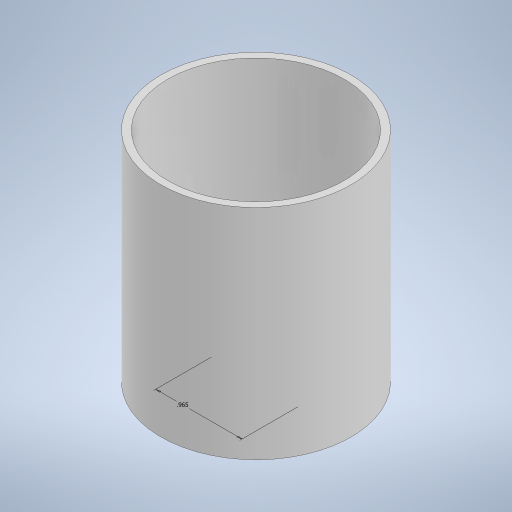
# Autodesk Inventor part: UpstreamVolume
Saved by Autodesk Inventor 2023 (Build 270158000, 158)
## iProperties
Created: 2023-01-27
Part Number: UpstreamVolume
Material: Generic
Document SubType Name: Modeling
Designer: remidm
Density: 1 g/cm^3
Appearance: Default
DistanceBetweenHolesSweep: 0.965 in
Author: remidm
Autodesk Inventor part; units mm, degrees
ref_plane "YZ Plane" through (0, 0, 0) normal (1, 0, 0) x (0, 1, 0)
ref_plane "XZ Plane" through (0, 0, 0) normal (0, 1, 0) x (-1, 0, 0)
ref_plane "XY Plane" through (0, 0, 0) normal (0, 0, 1) x (1, 0, 0)
sketch "Sketch1" plane through (0, 0, 0) normal (0, 0, 1) x (1, 0, 0)
  line L0 (-25, 0) -> (-25, 60)
  line L1 (-27, 60) -> (-27, -2)
  line L2 (-25, 0) -> (0, 0)
  line L3 (0, 0) -> (0, -2)
  line L4 (0, -2) -> (-27, -2)
  line L5 (0, -14.4) -> (0, 72.4) projected
  line L6 (-27, 60) -> (-25, 60)
  dimension "d5" = 2
  dimension "radius" = 25
  dimension "d7" = 2
  constraints: 12 end point, 2 horizontal, 2 perpendicular, 1 vertical
  measures "d5" distance between parallel lines of L4 L2
  measures "radius" distance from line of L2.end L0
  measures "d7" distance between parallel lines of L0 L1
revolve "Revolution1" add sketch "Sketch1" angle 360 about axis through (0, -10, 0) along (0, 1, 0)
sketch "Sketch3" plane through (0, -2, 0) normal (0, -1, 0) x (1, 0, 0)
  point P0 (0, 0)
  point P1 (-12.4915, 0)
  point P2 (12.0084, 0)
  dimension "DistanceBetweenHolesSweep" = 24.5
  measures "DistanceBetweenHolesSweep" distance of point (12.008, 0) point (-12.492, 0)
hole "Hole2" at (0, -2, 0) direction (0, 1, 0) diameter 5.08 end through all
hole "Hole3" at (-12.4915, -2, 0) at (12.0084, -2, 0) direction (0, 1, 0) diameter 5 end through all
equation "\"d22\" = fixation_holes_diameter"
equation "\"d30\" = PenetrationOuterDiameter"
equation "\"d5\" = thickness"
equation "\"radius\" = 0.5 * SaltDiameter"
equation "\"d7\" = thickness"
equation "\"thickness\" = crucible_thickness"
equation "\"fixation_holes_diameter\" = 5.08"
equation "\"PenetrationOuterDiameter\" = 5"
equation "\"SaltDiameter\" = 50"
equation "\"crucible_thickness\" = 2"
body "Solid1"
